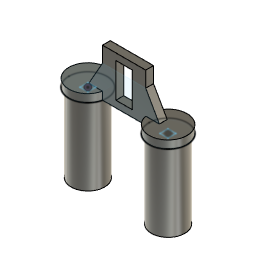
drzaknahrebenv1 (Autodesk Fusion 360 design; units mm, degrees)
Autodesk Fusion 360 part; units mm, degrees
note: some values were not read from the file. Chosen so that the rebuilt part matches the saved one: which bodies a step acts on.
sketch "Sketch1" plane through (0, 0, 0) normal (0, 0, 1) x (1, 0, 0)
  circle A0 centre (0, 0) radius 4.275
  line L0 (4.275, 0) -> (16.275, 0)
  circle A1 centre (20.55, 0) radius 4.275
  dimension "d1" = 8.55
  dimension "d3" = 12
  dimension "d4" = 8.55
  dimension "d5" = 4.275
  constraint coincident A0.centre origin
  constraint coincident A0 L0.start
  measures "d1" diameter of A0
  measures "d3" distance of L0.start L0.end
  measures "d4" diameter of A1
  measures "d5" distance of L0.end A1.centre
extrude "Extrude1" add sketch "Sketch1" against normal blind 20 makes body 1 at (24.8197, -0.2131, -13.3333) makes body 2 at (4.2697, -0.2131, -13.3333)
sketch "Sketch2" plane through (0, 0, 0) normal (0, 0, 1) x (-1, 0, 0)
  circle A0 centre (-20.55, 0) radius 4.275
  circle A1 centre (-20.55, 0) radius 4.85
  circle A2 centre (0, 0) radius 4.85
  line L0 (-1, -1) -> (1, -1)
  line L1 (1, -1) -> (1, 1)
  line L2 (1, 1) -> (-1, 1)
  line L3 (-1, 1) -> (-1, -1)
  line L4 (-21.5, 1) -> (-19.5, 1)
  line L5 (-19.5, 1) -> (-19.5, -1)
  line L6 (-19.5, -1) -> (-21.5, -1)
  line L7 (-21.5, -1) -> (-21.5, 1)
  dimension "d8" = 9.7
  dimension "d9" = 9.7
  constraint concentric A0 A1
  constraint coincident A2.centre origin
  constraint horizontal L0
  constraint vertical L1
  constraint horizontal L2
  constraint vertical L3
  constraint horizontal L4
  constraint vertical L5
  constraint horizontal L6
  constraint vertical L7
  measures "d8" diameter of A1
  measures "d9" diameter of A2
extrude "Extrude2" add sketch "Sketch2" along normal blind 2 contours L0 L1 L2 L3 | L4 L5 L6 L7 bodies 1 2
extrude "Extrude3" add 1 faces at (1, -0.3333, 0.6667) along direction (1, 0, 0) blind 20.5 on bodies 2 bodies 2 1
extrude "Extrude4" cut sketch "Sketch2" along normal blind 2 contours A0 | A1 | A2 bodies 2 makes body 3 at (24.8038, -0.4257, -6.6667) makes body 4 at (4.2538, -0.4257, -6.6667)
extrude "Extrude5" add sketch "Sketch2" along normal blind 2 contours A0 | A1 | A2 bodies 2 3 4
sketch "Sketch3" plane through (0, 0, 2) normal (0, 0, 1) x (-1, 0, 0)
  line L0 (-15.8042, -1) -> (-4.7458, -1)
  arc A0 (-4.7458, -1) -> (-4.7458, 1) centre (0, 0) ccw
  line L1 (-4.7458, 1) -> (-15.8042, 1)
  arc A1 (-15.8042, 1) -> (-15.8042, -1) centre (-20.55, 0) ccw
  line L2 (-4.7458, -1) -> (-15.8042, -1)
  line L3 (-15.8042, -1) -> (-15.8042, 1)
  line L4 (-15.8042, 1) -> (-4.7458, 1)
  line L5 (-4.7458, 1) -> (-4.7458, -1)
  constraint horizontal L2
  constraint vertical L3
  constraint horizontal L4
  constraint vertical L5
  constraint coincident L1.end A1.start
  constraint coincident L0.end A0.start
extrude "Extrude6" add sketch "Sketch3" along normal blind 6.2 contours L0 L1 L2 L3 L4 L5 bodies 2
sketch "Sketch4" plane through (0, 0, 2) normal (0, 0, 1) x (-1, 0, 0)
  line L0 (-4.7458, 1) -> (-4.7458, -1)
  arc A0 (-4.7458, -1) -> (-4.7458, 1) centre (0, 0) ccw
sketch "Sketch5" plane through (4.7458, 0, 0) normal (-1, 0, 0) x (0, -1, 0)
  line L0 (-1, 2) -> (1, 2)
  line L1 (1, 2) -> (1, 8.2)
  line L2 (1, 8.2) -> (-1, 8.2)
  line L3 (-1, 8.2) -> (-1, 2)
  line L4 (-1, 8.2) -> (1, 8.2)
  line L5 (1, 8.2) -> (1, 2)
  line L6 (1, 2) -> (-1, 2)
  line L7 (-1, 2) -> (-1, 8.2)
  constraint horizontal L4
  constraint vertical L5
  constraint horizontal L6
  constraint vertical L7
  constraint coincident L0.end L1.start
  constraint coincident L2.end L3.start
extrude "Extrude7" add sketch "Sketch5" along normal blind 3.5 bodies 2
sketch "Sketch6" plane through (0, 1, 0) normal (0, 1, 0) x (-1, 0, 0)
  line L0 (-15.8042, 2) -> (-15.8042, 0)
  line L1 (-15.8042, 0) -> (-4.7458, 0)
  line L2 (-4.7458, 0) -> (-4.7458, 2)
  line L3 (-4.7458, 2) -> (-1.2458, 2)
  line L4 (-1.2458, 2) -> (-1.2458, 8.2)
  line L5 (-1.2458, 8.2) -> (-15.8042, 8.2)
  line L6 (-15.8042, 8.2) -> (-15.8042, 2)
  line L7 (-1.2458, 2) -> (-4.7458, 8.2)
  constraint coincident L3.end L4.start
  constraint coincident L5 L7.end
extrude "Extrude8" cut sketch "Sketch6" against normal blind 2.5 contours L4 L5 L7 bodies 2
extrude "Extrude9" add 1 faces at (15.8042, -0.3333, 6.1333) along direction (1, 0, 0) blind 3.5 on bodies 2 bodies 2
sketch "Sketch7" plane through (0, 1, 0) normal (0, 1, 0) x (-1, 0, 0)
  line L0 (-1.2458, 2) -> (-4.7458, 8.2)
  line L1 (-4.7458, 8.2) -> (-19.3042, 8.2)
  line L2 (-19.3042, 8.2) -> (-19.3042, 2)
  line L3 (-19.3042, 2) -> (-15.8042, 2)
  line L4 (-15.8042, 2) -> (-15.8042, 0)
  line L5 (-15.8042, 0) -> (-4.7458, 0)
  line L6 (-4.7458, 0) -> (-4.7458, 2)
  line L7 (-4.7458, 2) -> (-1.2458, 2)
  line L8 (-19.3042, 2) -> (-15.8042, 8.2)
  constraint coincident L2.end L3.start
  constraint coincident L1 L8.end
extrude "Extrude10" cut sketch "Sketch7" against normal blind 2.5 contours L1 L2 L8 bodies 2
sketch "Sketch8" plane through (0, -1, 0) normal (0, -1, 0) x (1, 0, 0)
  line L0 (19.3042, 2) -> (15.8042, 8.2)
  line L1 (15.8042, 8.2) -> (4.7458, 8.2)
  line L2 (4.7458, 8.2) -> (1.2458, 2)
  line L3 (1.2458, 2) -> (4.7458, 2)
  line L4 (4.7458, 2) -> (4.7458, 0)
  line L5 (4.7458, 0) -> (15.8042, 0)
  line L6 (15.8042, 0) -> (15.8042, 2)
  line L7 (15.8042, 2) -> (19.3042, 2)
extrude "Extrude11" add 1 faces at (8.4319, 0.3333, 8.2) along direction (0, 0, 1) blind 4 on bodies 2 bodies 2
sketch "Sketch9" plane through (0, 1, 0) normal (0, 1, 0) x (-1, 0, 0)
  line L0 (-15.8042, 8.2) -> (-19.3042, 2)
  line L1 (-19.3042, 2) -> (-15.8042, 2)
  line L2 (-15.8042, 2) -> (-15.8042, 0)
  line L3 (-15.8042, 0) -> (-4.7458, 0)
  line L4 (-4.7458, 0) -> (-4.7458, 2)
  line L5 (-4.7458, 2) -> (-1.2458, 2)
  line L6 (-1.2458, 2) -> (-4.7458, 8.2)
  line L7 (-4.7458, 8.2) -> (-4.7458, 12.2)
  line L8 (-4.7458, 12.2) -> (-15.8042, 12.2)
  line L9 (-15.8042, 12.2) -> (-15.8042, 8.2)
  line L10 (-8.1748, 1.7) -> (-12.3748, 1.7)
  line L11 (-12.3748, 1.7) -> (-12.3748, 10.5)
  line L12 (-12.3748, 10.5) -> (-8.1748, 10.5)
  line L13 (-8.1748, 10.5) -> (-8.1748, 1.7)
  dimension "d30" = 4.2
  dimension "d31" = 8.8
  dimension "d32" = 3.429
  dimension "d33" = 1.7
  constraint horizontal L10
  constraint vertical L11
  constraint horizontal L12
  constraint vertical L13
  measures "d30" distance of L11 L13
  measures "d31" distance of L10 L12
  measures "d32" distance of L7 L13
  measures "d33" distance of L3 L10
extrude "Extrude12" cut sketch "Sketch9" against normal blind 2 contours L10 L11 L12 L13 bodies 2
sketch "Sketch10" plane through (0, -1, 0) normal (0, -1, 0) x (1, 0, 0)
equation "d18 = 8.2 mm - 2 mm"
